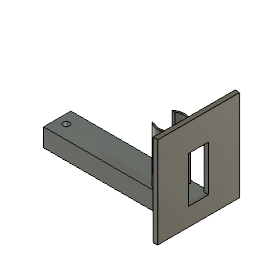
imaging_stand_assembly (Autodesk Fusion 360 archive; units mm, degrees)
design "写真撮影フォーム"
Autodesk Fusion 360 part; units mm, degrees
sketch "スケッチ1" plane through (0, 0, 0) normal (0, 0, 1) x (1, 0, 0)
  line L0 (75, -15) -> (-75, -15)
  line L1 (-75, -15) -> (-75, 15)
  line L2 (-75, 15) -> (75, 15)
  line L3 (75, 15) -> (75, -15)
  line L4 (75, -15) -> (-75, 15) construction
  line L5 (-75, -15) -> (75, 15) construction
  dimension "d1" = 150
  dimension "d2" = 30
  constraint horizontal L0
  constraint perpendicular L0 L1
  constraint parallel L0 L2
  constraint parallel L1 L3
  constraint coincident L4 origin
  constraint coincident L5 origin
  measures "d1" distance of L1.end L2.end
  measures "d2" distance of L0.end L1.end
extrude "押し出し1" add sketch "スケッチ1" along normal blind 20
sketch "スケッチ2" plane through (0, 0, 20) normal (0, 0, 1) x (-1, 0, 0)
  line L0 (-75, -15) -> (75, -15)
  line L1 (75, -15) -> (75, 15)
  line L2 (75, 15) -> (-75, 15)
  line L3 (-75, 15) -> (-75, -15)
sketch "スケッチ3" plane through (0, 0, 0) normal (0, 0, -1) x (1, 0, 0)
  line L0 (-75, -15) -> (75, -15)
  line L1 (75, -15) -> (75, 15)
  line L2 (75, 15) -> (-75, 15)
  line L3 (-75, 15) -> (-75, -15)
  circle A0 centre (-65, 0) radius 7.5
  dimension "d5" = 15
  measures "d5" diameter of A0
extrude "押し出し2" cut sketch "スケッチ3" against normal blind 15 contours A0
sketch "スケッチ4" plane through (0, 0, 15) normal (0, 0, -1) x (1, 0, 0)
  circle A0 centre (-65, 0) radius 7.5
  circle A1 centre (-65, 0) radius 3.5
  dimension "d8" = 7
  constraint concentric A0 A1
  measures "d8" diameter of A1
extrude "押し出し3" cut sketch "スケッチ4" against normal blind 10 contours A1
sketch "スケッチ5" plane through (0, 0, 20) normal (0, 0, 1) x (-1, 0, 0)
  circle A0 centre (-50, 0) radius 12
  dimension "d11" = 24
  measures "d11" diameter of A0
extrude "押し出し4" cut sketch "スケッチ5" against normal blind 2
sketch "スケッチ10" plane through (0, 0, 20) normal (0, 0, 1) x (-1, 0, 0)
  line L0 (-60, 15) -> (20, 15)
  line L1 (20, 15) -> (20, 20)
  line L2 (20, 20) -> (-60, 20)
  line L3 (-60, 20) -> (-60, 15)
  constraint horizontal L0
  constraint vertical L1
  constraint horizontal L2
  constraint vertical L3
sketch "スケッチ11" plane through (0, 0, 20) normal (0, 0, 1) x (-1, 0, 0)
  line L0 (-60, -15) -> (20, -15)
  line L1 (20, -15) -> (20, -20)
  line L2 (20, -20) -> (-60, -20)
  line L3 (-60, -20) -> (-60, -15)
  constraint horizontal L0
  constraint vertical L1
  constraint horizontal L2
  constraint vertical L3
sketch "スケッチ13" plane through (75, 0, 0) normal (1, 0, 0) x (0, 1, 0)
  line L0 (-15, 0) -> (15, 0)
  line L1 (15, 0) -> (15, 20)
  line L2 (15, 20) -> (-15, 20)
  line L3 (-15, 20) -> (-15, 0)
  line L4 (-44.8748, 0) -> (45.1252, 0)
  line L5 (45.1252, 0) -> (45.1252, 100)
  line L6 (45.1252, 100) -> (-44.8748, 100)
  line L7 (-44.8748, 100) -> (-44.8748, 0)
  dimension "d40" = 90
  constraint horizontal L4
  constraint vertical L5
  constraint horizontal L6
  constraint vertical L7
  measures "d40" distance of L5 L7
extrude "押し出し9" add sketch "スケッチ13" along normal blind 5
sketch "スケッチ14" plane through (80, 0, 0) normal (1, 0, 0) x (0, 1, 0)
  line L0 (-44.8748, 100) -> (-44.8748, 0)
  line L1 (-44.8748, 0) -> (45.1252, 0)
  line L2 (45.1252, 0) -> (45.1252, 100)
  line L3 (45.1252, 100) -> (-44.8748, 100)
  line L4 (-11, 20) -> (11, 20)
  line L5 (11, 20) -> (11, 70)
  line L6 (11, 70) -> (-11, 70)
  line L7 (-11, 70) -> (-11, 20)
  point P0 (0, 20)
  dimension "d28" = 22
  dimension "d29" = 50
  constraint horizontal L4
  constraint vertical L5
  constraint horizontal L6
  constraint vertical L7
  constraint midpoint L4 P0
  measures "d28" distance of L4.start L4.end
  measures "d29" distance of L4.start L6.end
extrude "押し出し10" cut sketch "スケッチ14" against normal blind 5 contours L4 L5 L6 L7
sketch "スケッチ15" plane through (0, 0, 20) normal (0, 0, 1) x (-1, 0, 0)
  circle A0 centre (-50, 0) radius 15
  circle A1 centre (-50, 0) radius 13
  dimension "d32" = 30
  dimension "d33" = 26
  constraint concentric A0 A1
  measures "d32" diameter of A0
  measures "d33" diameter of A1
extrude "押し出し11" add sketch "スケッチ15" along normal blind 60
sketch "スケッチ16" plane through (0, 0, 80) normal (0, 0, 1) x (-1, 0, 0)
  circle A0 centre (-50, 0) radius 13
  circle A1 centre (-50, 0) radius 15
  line L0 (-64.5, 11) -> (-35.5, 11)
  line L1 (-35.5, 11) -> (-35.5, -11)
  line L2 (-35.5, -11) -> (-64.5, -11)
  line L3 (-64.5, -11) -> (-64.5, 11)
  line L4 (-64.5, 11) -> (-35.5, -11) construction
  line L5 (-35.5, 11) -> (-64.5, -11) construction
  point P0 (-50, 0)
  dimension "d36" = 29
  dimension "d37" = 22
  constraint horizontal L0
  constraint perpendicular L0 L1
  constraint parallel L0 L2
  constraint parallel L1 L3
  constraint coincident L4 P0
  constraint coincident L5 P0
  constraint coincident P0 A0.centre
  measures "d36" distance of L1.end L2.end
  measures "d37" distance of L0.end L1.end
extrude "押し出し12" cut sketch "スケッチ16" against normal blind 60 contours A0 A1 L0 L1 L2 | A0 A1 L0 L2 L3 | A1 L1 | A1 L3
extrude "押し出し7" [rolled back] along distance -20 taper angle 0
sketch "スケッチ12" plane through (0, 0, 20) normal (0, 0, 1) x (-1, 0, 0)
  circle A0 centre (-60, 0) radius 12
  circle A1 centre (65, 0) radius 3.5
  line L0 (-75, -15) -> (-60, -15)
  line L1 (-60, -15) -> (-60, -20)
  line L2 (-60, -20) -> (20, -20)
  line L3 (20, -20) -> (20, -15)
  line L4 (20, -15) -> (75, -15)
  line L5 (75, -15) -> (75, 15)
  line L6 (75, 15) -> (20, 15)
  line L7 (20, 15) -> (20, 20)
  line L8 (20, 20) -> (-60, 20)
  line L9 (-60, 20) -> (-60, 15)
  line L10 (-60, 15) -> (-75, 15)
  line L11 (20, -20) -> (-60, -20)
  line L12 (-60, -20) -> (-60, -15)
  line L13 (-60, -15) -> (20, -15)
  line L14 (20, -15) -> (20, -20)
  line L15 (20, 20) -> (-60, 20)
  line L16 (-60, 20) -> (-60, 15)
  line L17 (-60, 15) -> (20, 15)
  line L18 (20, 15) -> (20, 20)
  arc A2 (-68.6603, -11) -> (-51.3397, -11) centre (-60, 0) ccw
  line L19 (-68.6603, -11) -> (-66.9282, -11)
  arc A3 (-66.9282, -11) -> (-53.0718, -11) centre (-60, 0) ccw
  line L20 (-53.0718, -11) -> (-51.3397, -11)
  line L21 (-75, 15) -> (-75, 11)
  line L22 (-75, 11) -> (-80, 11)
  line L23 (-80, 11) -> (-80, -11)
  line L24 (-80, -11) -> (-75, -11)
  line L25 (-75, -11) -> (-75, -15)
  line L26 (-51.3397, 11) -> (-53.0718, 11)
  arc A4 (-53.0718, 11) -> (-66.9282, 11) centre (-60, 0) ccw
  line L27 (-66.9282, 11) -> (-68.6603, 11)
  arc A5 (-51.3397, 11) -> (-68.6603, 11) centre (-60, 0) ccw
  constraint horizontal L11
  constraint vertical L12
  constraint horizontal L13
  constraint vertical L14
  constraint coincident L0.end L1.start
  constraint coincident L2.end L3.start
  constraint horizontal L15
  constraint vertical L16
  constraint horizontal L17
  constraint vertical L18
  constraint coincident L9.end L10.start
  constraint coincident L7.end L8.start
extrude "押し出し8" [rolled back] along distance 80 taper angle 0
sketch "スケッチ6" plane through (75, 0, 0) normal (1, 0, 0) x (0, 1, 0)
  line L0 (-15, 0) -> (15, 0)
  line L1 (15, 0) -> (15, 20)
  line L2 (15, 20) -> (-15, 20)
  line L3 (-15, 20) -> (-15, 0)
  line L4 (-25, 0) -> (25, 0)
  line L5 (25, 0) -> (25, 100)
  line L6 (25, 100) -> (-25, 100)
  line L7 (-25, 100) -> (-25, 0)
  dimension "d14" = 50
  dimension "d15" = 100
  constraint horizontal L4
  constraint vertical L5
  constraint horizontal L6
  constraint vertical L7
  constraint midpoint origin L4
  measures "d14" distance of L4.start L4.end
  measures "d15" distance of L4.start L6.end
extrude "押し出し5" [suppressed]
sketch "スケッチ8" plane through (75, 0, 0) normal (-1, 0, 0) x (0, -1, 0)
  line L0 (25, 0) -> (25, 100)
  line L1 (25, 100) -> (-25, 100)
  line L2 (-25, 100) -> (-25, 0)
  line L3 (-25, 0) -> (-15, 0)
  line L4 (-15, 0) -> (-15, 20)
  line L5 (-15, 20) -> (15, 20)
  line L6 (15, 20) -> (15, 0)
  line L7 (15, 0) -> (25, 0)
sketch "スケッチ9" plane through (75, 0, 0) normal (1, 0, 0) x (0, 1, 0)
  line L0 (-15, 0) -> (15, 0)
  line L1 (15, 0) -> (15, 20)
  line L2 (15, 20) -> (-15, 20)
  line L3 (-15, 20) -> (-15, 0)
  line L4 (-15, 20) -> (15, 20)
  line L5 (15, 20) -> (15, 70)
  line L6 (15, 70) -> (-15, 70)
  line L7 (-15, 70) -> (-15, 20)
  dimension "d18" = 30
  dimension "d19" = 50
  constraint horizontal L4
  constraint vertical L5
  constraint horizontal L6
  constraint vertical L7
  constraint coincident L2.end L3.start
  measures "d18" distance of L2.end L1.end
  measures "d19" distance of L2.end L6.end
extrude "押し出し6" [suppressed]

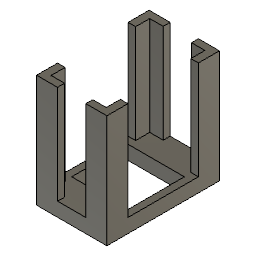
design "照明固定器具"
Autodesk Fusion 360 part; units mm, degrees
sketch "スケッチ1" plane through (0, 0, 0) normal (0, 0, 1) x (1, 0, 0)
  line L0 (25, -40) -> (-25, -40)
  line L1 (-25, -40) -> (-25, 40)
  line L2 (-25, 40) -> (25, 40)
  line L3 (25, 40) -> (25, -40)
  line L4 (25, -40) -> (-25, 40) construction
  line L5 (-25, -40) -> (25, 40) construction
  dimension "d1" = 50
  dimension "d2" = 80
  constraint horizontal L0
  constraint perpendicular L0 L1
  constraint parallel L0 L2
  constraint parallel L1 L3
  constraint coincident L4 origin
  constraint coincident L5 origin
  measures "d1" distance of L1.end L2.end
  measures "d2" distance of L0.end L1.end
extrude "押し出し1" add sketch "スケッチ1" along normal blind 80
sketch "スケッチ2" plane through (0, 0, 80) normal (0, 0, 1) x (-1, 0, 0)
  line L0 (-25, -40) -> (25, -40)
  line L1 (25, -40) -> (25, 40)
  line L2 (25, 40) -> (-25, 40)
  line L3 (-25, 40) -> (-25, -40)
  line L4 (-19.6, 35) -> (19.6, 35)
  line L5 (19.6, 35) -> (19.6, -35)
  line L6 (19.6, -35) -> (-19.6, -35)
  line L7 (-19.6, -35) -> (-19.6, 35)
  line L8 (-19.6, 35) -> (19.6, -35) construction
  line L9 (19.6, 35) -> (-19.6, -35) construction
  dimension "d5" = 39.2
  dimension "d6" = 70
  constraint horizontal L4
  constraint perpendicular L4 L5
  constraint parallel L4 L6
  constraint parallel L5 L7
  constraint coincident L8 origin
  constraint coincident L9 origin
  measures "d5" distance of L5.end L6.end
  measures "d6" distance of L4.end L5.end
extrude "押し出し2" cut sketch "スケッチ2" against normal blind 70 contours L4 L5 L6 L7
sketch "スケッチ4" plane through (0, 0, 80) normal (0, 0, 1) x (-1, 0, 0)
  line L0 (19.6, 35) -> (19.6, -35)
  line L1 (19.6, -35) -> (-19.6, -35)
  line L2 (-19.6, -35) -> (-19.6, 35)
  line L3 (-19.6, 35) -> (19.6, 35)
  line L4 (-25, -40) -> (25, -40)
  line L5 (25, -40) -> (25, 40)
  line L6 (25, 40) -> (-25, 40)
  line L7 (-25, 40) -> (-25, -40)
  line L8 (-30, 25) -> (30, 25)
  line L9 (30, 25) -> (30, -25)
  line L10 (30, -25) -> (-30, -25)
  line L11 (-30, -25) -> (-30, 25)
  line L12 (-30, 25) -> (30, -25) construction
  line L13 (30, 25) -> (-30, -25) construction
  dimension "d11" = 60
  dimension "d12" = 50
  constraint horizontal L8
  constraint perpendicular L8 L9
  constraint parallel L8 L10
  constraint parallel L9 L11
  constraint coincident L12 origin
  constraint coincident L13 origin
  measures "d11" distance of L9.end L10.end
  measures "d12" distance of L8.end L9.end
extrude "押し出し4" cut sketch "スケッチ4" against normal blind 70 contours L0 L5 L8 L10 | L2 L7 L8 L10
sketch "スケッチ5" plane through (0, 0, 10) normal (0, 0, 1) x (-1, 0, 0)
  line L0 (-19.6, -35) -> (19.6, -35)
  line L1 (19.6, -35) -> (19.6, -25)
  line L2 (19.6, -25) -> (25, -25)
  line L3 (25, -25) -> (25, 25)
  line L4 (25, 25) -> (19.6, 25)
  line L5 (19.6, 25) -> (19.6, 35)
  line L6 (19.6, 35) -> (-19.6, 35)
  line L7 (-19.6, 35) -> (-19.6, 25)
  line L8 (-19.6, 25) -> (-25, 25)
  line L9 (-25, 25) -> (-25, -25)
  line L10 (-25, -25) -> (-19.6, -25)
  line L11 (-19.6, -25) -> (-19.6, -35)
  line L12 (-20, 20) -> (20, 20)
  line L13 (20, 20) -> (20, -20)
  line L14 (20, -20) -> (-20, -20)
  line L15 (-20, -20) -> (-20, 20)
  line L16 (-20, 20) -> (20, -20) construction
  line L17 (20, 20) -> (-20, -20) construction
  constraint horizontal L12
  constraint perpendicular L12 L13
  constraint parallel L12 L14
  constraint parallel L13 L15
  constraint coincident L16 origin
  constraint coincident L17 origin
extrude "押し出し5" cut sketch "スケッチ5" against normal blind 10 contours L12 L13 L14 L15
sketch "スケッチ6" plane through (0, -40, 0) normal (0, -1, 0) x (1, 0, 0)
  line L0 (-25, 0) -> (25, 0)
  line L1 (25, 0) -> (25, 80)
  line L2 (25, 80) -> (-25, 80)
  line L3 (-25, 80) -> (-25, 0)
  line L4 (-10, 80) -> (10, 80)
  line L5 (10, 80) -> (10, 10)
  line L6 (10, 10) -> (-10, 10)
  line L7 (-10, 10) -> (-10, 80)
  constraint horizontal L4
  constraint vertical L5
  constraint horizontal L6
  constraint vertical L7
  constraint coincident L2 L4.start
extrude "押し出し6" cut sketch "スケッチ6" against normal blind 100 contours L2 L4 L5 L6 L7
